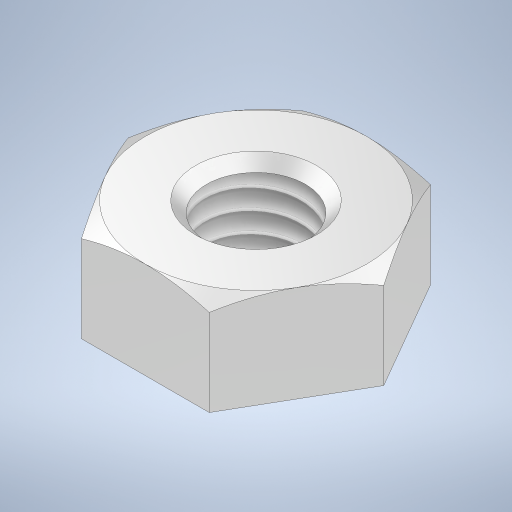
# Autodesk Inventor part: UNT-03
Saved by Autodesk Inventor 2024.2 (Build 282272000, 272)
## iProperties
Part Number: UNT-03
Material: Stainless Steel AISI 304
Document SubType Name: Modeling
Designer: Masato Kubotera
Density: 8 g/cm^3
Appearance: Chrome - Satin
Catalog Web Link: https://wilco.jp/products/U/UNT-3.html
Mass: 0.301111 g
Surface Area: 0.863829 cm^2
Volume: 0.0376389 cm^3
Author: Masato Kubotera
Autodesk Inventor part; units mm, degrees
ref_plane "YZ Plane" through (0, 0, 0) normal (1, 0, 0) x (0, 1, 0)
ref_plane "XZ Plane" through (0, 0, 0) normal (0, 1, 0) x (-1, 0, 0)
ref_plane "XY Plane" through (0, 0, 0) normal (0, 0, 1) x (1, 0, 0)
sketch "Sketch1" plane through (0, 0, 0) normal (0, 1, 0) x (-1, 0, 0)
  line L0 (0, 1.2) -> (0, -1.2)
  line L1 (0, -1.2) -> (-3.1754, -1.2)
  line L2 (-3.1754, -1.2) -> (-3.1754, 0.9544)
  line L3 (-2.75, 1.2) -> (0, 1.2)
  line L4 (-2.75, 1.2) -> (-3.1754, 0.9544)
  line L5 (0, 0) -> (-3.1754, 0) construction
  dimension "d0" = 2.4
  dimension "d1" = 5.5
  dimension "d2" = 6.3509
  dimension "d3" = 30
  constraints: 12 end point, 3 horizontal, 2 vertical, 1 coincident, 1 midpoint
  measures "d0" distance of L0.start L0.end
  measures "d1" diameter of L3.start L0
  measures "d2" diameter of L2 L0
  measures "d3" angle of L3 L4
revolve "Revolution1" add sketch "Sketch1" angle 360 about axis through (0, 0, 1.2) along (0, 0, -1)
sketch "Sketch2" plane through (0, 0, 1.2) normal (0, 0, 1) x (1, 0, 0)
  circle A0 centre (0, 0) radius 3.1754 projected
  line L0 (0, 3.1754) -> (2.75, 1.5877)
  line L1 (2.75, 1.5877) -> (2.75, -1.5877)
  line L2 (2.75, -1.5877) -> (0, -3.1754)
  line L3 (0, -3.1754) -> (-2.75, -1.5877)
  line L4 (-2.75, -1.5877) -> (-2.75, 1.5877)
  line L5 (-2.75, 1.5877) -> (0, 3.1754)
  point P0 (0, 0)
  point P1 (0, 0)
  point P2 (0, 0)
  point P3 (-2.75, -1.5877)
  point P4 (-2.75, -1.5877)
  point P5 (0, -3.1754)
  point P6 (0, -3.1754)
  constraints: 12 end point, 2 coincident, 1 vertical, 15 other
extrude "Extrusion1" cut sketch "Sketch2" against normal through all contours A0 L1 | L0 A0 | A0 L2 | L5 A0 | A0 L3 | L4 A0
hole "Hole1" at (0, 0, 1.2) direction (0, 0, -1) diameter 2.459 depth 6 countersink diameter 3 countersink angle 90 thread size "M3x0.5" class "6H" standard "ANSI Metric M Profile"
mirror "Mirror1" about plane through (0, 0, 0) normal (0, 0, 1) of "Hole1"
equation "\"d2\" = 1.1547 * d1"
body "Solid1"
